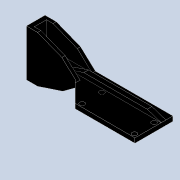
# Autodesk Inventor part: Y Axis Limit Switch Mount
Saved by Autodesk Inventor 2022 (Build 260153000, 153)
## iProperties
Created: 2021-10-29
Part Number: Y Axis Limit Switch Mount
Material: Generic
Document SubType Name: Modeling
Designer: Coy
Density: 1 g/cm^3
Appearance: Anodized - Black
Author: Coy
Autodesk Inventor part; units mm, degrees
ref_plane "YZ Plane" through (0, 0, 0) normal (1, 0, 0) x (0, 1, 0)
ref_plane "XZ Plane" through (0, 0, 0) normal (0, 1, 0) x (-1, 0, 0)
ref_plane "XY Plane" through (0, 0, 0) normal (0, 0, 1) x (1, 0, 0)
sketch "Sketch1" plane through (0, 0, 0) normal (1, 0, 0) x (0, 1, 0)
  line L0 (0, 0) -> (50, 0)
  line L1 (50, 0) -> (50, 20)
  line L2 (50, 20) -> (0, 20)
  line L3 (0, 20) -> (0, 0)
  dimension "d0" = 50
  dimension "d1" = 20
  constraints: 8 end point, 2 parallel, 1 horizontal, 1 perpendicular
  measures "d0" distance of L2.end L1.end
  measures "d1" distance of L1.end L0.end
extrude "Extrusion1" add sketch "Sketch1" along normal blind 5
sketch "Sketch2" plane through (5, 0, 0) normal (1, 0, 0) x (0, 0, -1)
  line L0 (-20, 50) -> (-20, 0) projected
  line L1 (-20, 25) -> (0, 25)
  line L2 (0, 0) -> (0, 50) projected
  line L3 (-20, 20) -> (0, 20)
  line L4 (0, 50) -> (-20, 50) construction
  line L5 (-10, 50) -> (-10, 0) construction
  line L6 (-20, 0) -> (0, 0) construction
  circle A0 centre (-10, 37.5) radius 2.6
  circle A1 centre (-10, 12.5) radius 2.6
  circle A2 centre (-10, 37.5) radius 4.625 construction
  circle A3 centre (-10, 12.5) radius 4.625 construction
  line L7 (-20, 25) -> (-16.5, 25)
  line L8 (-16.5, 25) -> (-16.5, 50)
  line L9 (-16.5, 50) -> (-20, 50)
  line L10 (-20, 50) -> (-20, 25)
  line L11 (0, 25) -> (-3.5, 25)
  line L12 (-3.5, 25) -> (-3.5, 50)
  line L13 (-3.5, 50) -> (0, 50)
  line L14 (0, 50) -> (0, 25)
  line L15 (-20, 20) -> (-16.5, 20)
  line L16 (-16.5, 20) -> (-16.5, 0)
  line L17 (-16.5, 0) -> (-20, 0)
  line L18 (-20, 0) -> (-20, 20)
  line L19 (0, 20) -> (-3.5, 20)
  line L20 (-3.5, 20) -> (-3.5, 0)
  line L21 (-3.5, 0) -> (0, 0)
  line L22 (0, 0) -> (0, 20)
  dimension "d4" = 5
  dimension "d5" = 5.2
  dimension "d6" = 5.2
  dimension "d7" = 12.5
  dimension "d8" = 12.5
  dimension "d9" = 9.25
  dimension "d10" = 9.25
  dimension "d11" = 3.5
  dimension "d12" = 3.5
  dimension "d13" = 3.5
  dimension "d14" = 3.5
  constraints: 38 end point, 9 parallel, 6 point on line, 4 centre point, 4 horizontal, 4 midpoint, 4 perpendicular, 2 coincident
  measures "d4" distance between parallel lines of L1 L3
  measures "d5" diameter of A0
  measures "d6" diameter of A1
  measures "d7" distance from line of L4 A0.centre
  measures "d8" distance from line of L6 A1.centre
  measures "d9" diameter of A2
  measures "d10" diameter of A3
  measures "d11" distance of L9.end L8.end
  measures "d12" distance of L12.end L13.end
  measures "d13" distance of L16.end L17.end
  measures "d14" distance of L21.end L20.end
extrude "Extrusion2" add sketch "Sketch2" along normal blind 49 contours L9 L8 L1 L0 | L1 L2 L3 L0 | L3 L16 L17 L0 | L12 L13 L2 L1 | L3 L2 L21 L20
chamfer "Chamfer1" distance 25 distance2 27 1 edges at (54, 50, 1.75) measured on face at (54, 23.3333, 18.8333)
chamfer "Chamfer2" distance 25 distance2 27 1 edges at (54, 50, 18.25) measured on face at (54, 23.3333, 18.8333)
chamfer "Chamfer3" distance 20 distance2 27 1 edges at (54, 0, 18.25) measured on face at (54, 15, 18.8333)
chamfer "Chamfer4" distance 20 distance2 27 1 edges at (54, 0, 1.75) measured on face at (54, 15, 1.1667)
sketch "Sketch3" plane through (54, 0, 0) normal (1, 0, 0) x (0, 0, -1)
  line L0 (0, 20) -> (-3.5, 20) projected
  line L1 (0, 20) -> (0, 25) projected
  line L2 (-3.5, 25) -> (0, 25) projected
  line L3 (-3.5, 25) -> (-16.5, 25) projected
  line L4 (-20, 25) -> (-16.5, 25) projected
  line L5 (-20, 25) -> (-20, 20) projected
  line L6 (-16.5, 20) -> (-20, 20) projected
  line L7 (-16.5, 20) -> (-3.5, 20) projected
  point P0 (0, 0)
extrude "Extrusion3" add sketch "Sketch3" along normal blind 83
sketch "Sketch4" plane through (5, 25, 16.5) normal (0, 1, 0) x (1, 0, 0)
  line L0 (132, -3.5) -> (132, 16.5) projected
  line L1 (132, 9) -> (34, 9)
  line L2 (34, 9) -> (34, 4)
  line L3 (34, 4) -> (132, 4)
  line L4 (132, 4) -> (132, 9)
  line L5 (49, 16.5) -> (132, 16.5) projected
  point P0 (-5, 16.5)
  dimension "d31" = 98
  dimension "d32" = 5
  dimension "d33" = 7.5
  constraints: 8 end point, 2 parallel, 1 horizontal, 1 perpendicular, 1 point on line
  measures "d31" distance of L3.end L2.end
  measures "d32" distance of L2.end L1.end
  measures "d33" distance between parallel lines of L5 L1
extrude "Extrusion4" add sketch "Sketch4" along normal blind 5
sketch "Sketch5" plane through (5, 20, 3.5) normal (0, -1, 0) x (1, 0, 0)
  line L0 (34, 9) -> (34, 4) projected
  line L1 (132, 9) -> (34, 9) projected
  line L2 (34, 4) -> (132, 4) projected
  line L3 (132, 16.5) -> (132, -3.5) projected
  point P0 (-5, -3.5)
extrude "Extrusion5" add sketch "Sketch5" along normal blind 5
chamfer "Chamfer5" distance 15 distance2 5 1 edges at (137, 30, 10) measured on face at (104.3333, 30, 10.8333)
chamfer "Chamfer6" distance 15 distance2 5 1 edges at (39, 30, 10) measured on face at (94.3333, 30, 10.8333)
chamfer "Chamfer7" distance 15 distance2 5 1 edges at (137, 15, 10) measured on face at (104.3333, 15, 9.1667)
chamfer "Chamfer8" distance 15 distance2 5 1 edges at (39, 15, 10) measured on face at (94.3333, 15, 9.1667)
sketch "Sketch6" plane through (5, 0, 0) normal (1, 0, 0) x (0, 0, -1)
  line L0 (-3.5, 50) -> (-16.5, 50) construction
  line L1 (-10, 50) -> (-10, 0) construction
  line L2 (-20, 0) -> (0, 0) construction
  circle A0 centre (-10, 37.5) radius 2.6
  circle A1 centre (-10, 12.5) radius 2.6
  dimension "d50" = 5.2
  dimension "d51" = 5.2
  dimension "d52" = 12.5
  dimension "d53" = 12.5
  constraints: 2 centre point, 2 end point, 2 midpoint, 2 point on line
  measures "d50" diameter of A0
  measures "d51" diameter of A1
  measures "d52" distance from line of L0 A0.centre
  measures "d53" distance from line of L2 A1.centre
extrude "Extrusion6" cut sketch "Sketch6" against normal up to next
sketch "Sketch7" plane through (0, 0, 20) normal (0, 0, 1) x (1, 0, 0)
  line L0 (39, 20) -> (137, 20) projected
  line L1 (39, 25) -> (137, 25) projected
  line L2 (137, 20) -> (73, 20)
  line L3 (73, 20) -> (73, 25)
  line L4 (73, 25) -> (137, 25)
  line L5 (137, 25) -> (137, 20)
  point P0 (0, 0)
  point P1 (73, 20)
  dimension "d56" = 64
  constraints: 8 end point, 2 parallel, 1 horizontal, 1 perpendicular, 1 point on line
  measures "d56" distance of L3.end L4.end
extrude "Extrusion7" add sketch "Sketch7" along normal blind 20.7
sketch "Sketch8" plane through (5, 25, 16.5) normal (0, 1, 0) x (1, 0, 0)
  line L0 (68, -3.5) -> (68, -24.2) projected
  line L1 (68, -24.2) -> (132, -24.2)
  line L2 (132, -24.2) -> (132, 3.8)
  line L3 (132, 3.8) -> (68, 3.8)
  line L4 (68, 3.8) -> (68, -24.2)
  line L5 (72, -20.7) -> (128, -20.7) construction
  line L6 (128, -20.7) -> (128, 0.3) construction
  line L7 (128, 0.3) -> (72, 0.3) construction
  line L8 (72, 0.3) -> (72, -20.7) construction
  circle A0 centre (72, -20.7) radius 2.6
  circle A1 centre (72, 0.3) radius 2.6
  circle A2 centre (128, -20.7) radius 2.6
  circle A3 centre (128, 0.3) radius 2.6
  point P0 (-5, 16.5)
  dimension "d59" = 64
  dimension "d60" = 28
  dimension "d61" = 56
  dimension "d62" = 21
  dimension "d63" = 3.5
  dimension "d64" = 4
  dimension "d65" = 5.2
  dimension "d66" = 5.2
  dimension "d67" = 5.2
  dimension "d68" = 5.2
  constraints: 16 end point, 4 centre point, 4 coincident, 4 parallel, 2 horizontal, 2 perpendicular
  measures "d59" distance of L3.end L2.end
  measures "d60" distance of L2.end L1.end
  measures "d61" distance of L7.end L6.end
  measures "d62" distance of L6.end L5.end
  measures "d63" distance between parallel lines of L1 L5
  measures "d64" distance between parallel lines of L0 L8
  measures "d65" diameter of A0
  measures "d66" diameter of A1
  measures "d67" diameter of A2
  measures "d68" diameter of A3
extrude "Extrusion8" cut sketch "Sketch8" against normal up to next contours A0 | A1 | A2 | A3
sketch "Sketch9" plane through (5, 20, 3.5) normal (0, -1, 0) x (1, 0, 0)
  line L0 (68, 37.2) -> (132, 37.2) projected
  line L1 (117, 9) -> (49, 9) projected
  line L2 (102.5, 37.2) -> (97.5, 37.2)
  line L3 (97.5, 37.2) -> (97.5, 9)
  line L4 (97.5, 9) -> (102.5, 9)
  line L5 (102.5, 9) -> (102.5, 37.2)
  line L6 (132, 9) -> (132, 37.2) projected
  point P0 (-5, -3.5)
  point P1 (102.5, 9)
  dimension "d71" = 5
  dimension "d72" = 29.5
  constraints: 8 end point, 2 parallel, 2 point on line, 1 horizontal, 1 perpendicular
  measures "d71" distance of L4.end L3.end
  measures "d72" distance between parallel lines of L6 L5
extrude "Extrusion9" add sketch "Sketch9" along normal blind 5
chamfer "Chamfer9" distance 15 distance2 5 1 edges at (105, 15, 40.7) measured on face at (92.8333, 15, 9.1667)
chamfer "Chamfer10" distance 15 angle 45 4 edges at (27, 50, 18.25) (27, 50, 1.75) (27, 0, 1.75) (27, 0, 18.25)
chamfer "Chamfer11" distance 20.7 angle 45 1 edges at (73, 22.5, 20)
equation "\"d8\" = d7"
equation "\"d10\" = d9"
equation "\"d53\" = d52"
equation "\"d54\" = d51"
body "Solid1"
